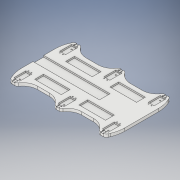
# Autodesk Inventor part: Body_Top
Saved by Autodesk Inventor 2017 (Build 210142000, 142)
## iProperties
Created: 2017-01-25
Part Number: Body_Top
Material: PVC, Unplasticized
Document SubType Name: Modeling
Designer: Alexander Miller
Density: 1.29 g/cm^3
Appearance: Smooth - White
material_thickness: 5,000 mm
body_width: 165,000 mm
leg_distance: 120,000 mm
Author: Alexander Miller
Autodesk Inventor part; units mm, degrees
ref_plane "YZ Plane" through (0, 0, 0) normal (1, 0, 0) x (0, 1, 0)
ref_plane "XZ Plane" through (0, 0, 0) normal (0, 1, 0) x (-1, 0, 0)
ref_plane "XY Plane" through (0, 0, 0) normal (0, 0, 1) x (1, 0, 0)
sketch "Sketch1" plane through (0, 0, 0) normal (0, 1, 0) x (-1, 0, 0)
  line L0 (-175, 0) -> (-175, -82.5)
  line L1 (-175, -82.5) -> (-165, -82.5)
  line L2 (-165, -82.5) -> (-165, -109.25)
  line L3 (-165, -109.25) -> (-135, -109.25)
  line L4 (-135, -109.25) -> (-135, -82.5)
  line L5 (-135, -82.5) -> (-15, -82.5)
  line L6 (-15, -82.5) -> (-15, -109.25)
  line L7 (-15, -109.25) -> (15, -109.25)
  line L8 (15, -109.25) -> (15, -82.5)
  line L9 (15, -82.5) -> (135, -82.5)
  line L10 (135, -82.5) -> (135, -109.25)
  line L11 (135, -109.25) -> (165, -109.25)
  line L12 (165, -109.25) -> (165, -82.5)
  line L13 (165, -82.5) -> (175, -82.5)
  line L14 (175, -82.5) -> (175, 0)
  line L15 (245, 0) -> (-245, 0) projected
  line L16 (-175, 0) -> (-175, 82.5)
  line L17 (-175, 82.5) -> (-165, 82.5)
  line L18 (-165, 82.5) -> (-165, 109.25)
  line L19 (-165, 109.25) -> (-135, 109.25)
  line L20 (-135, 109.25) -> (-135, 82.5)
  line L21 (-135, 82.5) -> (-15, 82.5)
  line L22 (-15, 82.5) -> (-15, 109.25)
  line L23 (-15, 109.25) -> (15, 109.25)
  line L24 (15, 109.25) -> (15, 82.5)
  line L25 (15, 82.5) -> (135, 82.5)
  line L26 (135, 82.5) -> (135, 109.25)
  line L27 (135, 109.25) -> (165, 109.25)
  line L28 (165, 109.25) -> (165, 82.5)
  line L29 (165, 82.5) -> (175, 82.5)
  line L30 (175, 82.5) -> (175, 0)
  point P0 (0, 0)
  point P1 (0, -109.25)
  dimension "d0" = 30
  dimension "d1" = 82.5
  dimension "d2" = 26.75
  dimension "d3" = 10
  dimension "d4" = 120
  constraints: 60 end point, 18 point on line, 14 symmetric about line, 9 perpendicular, 5 equal length, 2 vertical, 1 horizontal alignment, 1 midpoint, 1 vertical alignment
  measures "d0" distance of L10.end L11.end
  measures "d1" distance of L13.end L14.end
  measures "d2" distance of L11.end L12.end
  measures "d3" distance of L12.end L13.end
  measures "d4" distance of L8.end L9.end
extrude "Extrusion1" add sketch "Sketch1" along normal blind 10
sketch "Sketch2" plane through (0, 10, 0) normal (0, 1, 0) x (1, 0, 0)
  line L0 (-140, 57.25) -> (-160, 57.25)
  line L1 (-160, 57.25) -> (-160, 97.75)
  line L2 (-160, 97.75) -> (-140, 97.75)
  line L3 (-140, 97.75) -> (-140, 57.25)
  line L4 (10, 57.25) -> (-10, 57.25)
  line L5 (-10, 57.25) -> (-10, 97.75)
  line L6 (-10, 97.75) -> (10, 97.75)
  line L7 (10, 97.75) -> (10, 57.25)
  line L8 (160, 57.25) -> (140, 57.25)
  line L9 (140, 57.25) -> (140, 97.75)
  line L10 (140, 97.75) -> (160, 97.75)
  line L11 (160, 97.75) -> (160, 57.25)
  line L12 (-245, 0) -> (245, 0) projected
  line L13 (-140, -57.25) -> (-160, -57.25)
  line L14 (-160, -57.25) -> (-160, -97.75)
  line L15 (-160, -97.75) -> (-140, -97.75)
  line L16 (-140, -97.75) -> (-140, -57.25)
  line L17 (10, -57.25) -> (-10, -57.25)
  line L18 (-10, -57.25) -> (-10, -97.75)
  line L19 (-10, -97.75) -> (10, -97.75)
  line L20 (10, -97.75) -> (10, -57.25)
  line L21 (160, -57.25) -> (140, -57.25)
  line L22 (140, -57.25) -> (140, -97.75)
  line L23 (140, -97.75) -> (160, -97.75)
  line L24 (160, -97.75) -> (160, -57.25)
  line L25 (-135, 109.25) -> (-165, 109.25) projected
  line L26 (-165, 109.25) -> (-165, 82.5) projected
  line L27 (-15, 109.25) -> (-15, 82.5) projected
  line L28 (135, 109.25) -> (135, 82.5) projected
  point P0 (0, 0)
  dimension "d7" = 11.5
  dimension "d8" = 5
  dimension "d9" = 20
  dimension "d10" = 40.5
  dimension "d11" = 5
  dimension "d12" = 5
  constraints: 48 end point, 12 symmetric about line, 6 parallel, 4 point on line, 3 horizontal, 3 perpendicular, 2 collinear, 2 horizontal alignment
  measures "d7" distance between parallel lines of L2 L25
  measures "d8" distance between parallel lines of L1 L26
  measures "d9" distance of L1.end L2.end
  measures "d10" distance of L2.end L0.start
  measures "d11" distance between parallel lines of L27 L5
  measures "d12" distance between parallel lines of L9 L28
extrude "Extrusion2" cut sketch "Sketch2" against normal blind 5
sketch "Sketch3" plane through (0, 10, 0) normal (0, 1, 0) x (1, 0, 0)
  circle A0 centre (-155, 53.25) radius 2.25 construction
  circle A1 centre (-145, 53.25) radius 2.25 construction
  circle A2 centre (-155, 101.75) radius 2.25 construction
  circle A3 centre (-145, 101.75) radius 2.25 construction
  circle A4 centre (-5, 53.25) radius 2.25 construction
  circle A5 centre (-5, 101.75) radius 2.25 construction
  line L0 (-135, 109.25) -> (-165, 109.25) projected
  line L1 (-160, 97.75) -> (-140, 97.75) projected
  line L2 (-140, 57.25) -> (-160, 57.25) projected
  line L3 (-160, 57.25) -> (-160, 97.75) projected
  line L4 (-140, 97.75) -> (-140, 57.25) projected
  line L5 (-10, 57.25) -> (-10, 97.75) projected
  line L6 (-245, 0) -> (245, 0) projected
  line L7 (0, 152.95) -> (0, -152.95) projected
  circle A6 centre (-155, 53.25) radius 1.5
  circle A7 centre (-145, 53.25) radius 1.5
  circle A8 centre (-155, 101.75) radius 1.5
  circle A9 centre (-145, 101.75) radius 1.5
  circle A10 centre (-5, 53.25) radius 1.5
  circle A11 centre (-5, 101.75) radius 1.5
  circle A12 centre (155, 53.25) radius 1.5
  circle A13 centre (145, 53.25) radius 1.5
  circle A14 centre (155, 101.75) radius 1.5
  circle A15 centre (145, 101.75) radius 1.5
  circle A16 centre (5, 53.25) radius 1.5
  circle A17 centre (5, 101.75) radius 1.5
  circle A18 centre (-155, -53.25) radius 1.5
  circle A19 centre (-145, -53.25) radius 1.5
  circle A20 centre (-155, -101.75) radius 1.5
  circle A21 centre (-145, -101.75) radius 1.5
  circle A22 centre (-5, -53.25) radius 1.5
  circle A23 centre (-5, -101.75) radius 1.5
  circle A24 centre (155, -53.25) radius 1.5
  circle A25 centre (145, -53.25) radius 1.5
  circle A26 centre (155, -101.75) radius 1.5
  circle A27 centre (145, -101.75) radius 1.5
  circle A28 centre (5, -53.25) radius 1.5
  circle A29 centre (5, -101.75) radius 1.5
  point P0 (0, 0)
  dimension "d17" = 4
  dimension "d18" = 4
  dimension "d19" = 4.5
  dimension "d25" = 2.75
  dimension "d26" = 2.75
  dimension "d27" = 2.75
  dimension "d70" = 3
  constraints: 30 centre point, 18 symmetric about line, 10 equal radius, 6 concentric, 4 horizontal alignment, 3 vertical alignment, 18 other
  measures "d17" distance from line of L1 A2.centre
  measures "d18" distance from line of L2 A0.centre
  measures "d19" diameter of A2
  measures "d25" distance edge to line of A2 L3
  measures "d26" distance edge to line of A3 L4
  measures "d27" distance edge to line of A5 L5
  measures "d70" diameter of A8
extrude "Extrusion3" cut sketch "Sketch3" against normal through all contours A6 | A7 | A8 | A9 | A10 | A11 | A12 | A13 | A14 | A15 | A16 | A17 | A18 | A19 | A20 | A21 | A22 | A23 | A24 | A25 | A26 | A27 | A28 | A29
fillet "Fillet1" radius 10 12 edges at (-165, 5, 109.25) (-135, 5, 109.25) (-15, 5, 109.25) (15, 5, 109.25) (135, 5, 109.25) (165, 5, 109.25) (165, 5, -109.25) (135, 5, -109.25) (15, 5, -109.25) (-15, 5, -109.25) (-135, 5, -109.25) (-165, 5, -109.25)
fillet "Fillet2" radius 50 8 edges at (-135, 5, 82.5) (-15, 5, 82.5) (15, 5, 82.5) (135, 5, 82.5) (135, 5, -82.5) (15, 5, -82.5) (-15, 5, -82.5) (-135, 5, -82.5)
fillet "Fillet3" radius 100 8 edges at (-175, 5, 82.5) (-165, 5, 82.5) (165, 5, 82.5) (175, 5, 82.5) (175, 5, -82.5) (165, 5, -82.5) (-165, 5, -82.5) (-175, 5, -82.5)
sketch "Sketch10" plane through (0, 0, 0) normal (0, -1, 0) x (1, 0, 0)
  circle A0 centre (-150, 87.75) radius 2
  circle A1 centre (0, 87.75) radius 2
  circle A2 centre (150, 87.75) radius 2
  line L0 (-140, 97.75) -> (-160, 97.75) projected
  line L1 (10, 97.75) -> (-10, 97.75) projected
  line L2 (160, 97.75) -> (140, 97.75) projected
  line L3 (-245, 0) -> (245, 0) projected
  circle A3 centre (-150, -87.75) radius 2
  circle A4 centre (0, -87.75) radius 2
  circle A5 centre (150, -87.75) radius 2
  point P0 (0, 0)
  point P1 (-150, 97.75)
  point P2 (0, 97.75)
  point P3 (150, 97.75)
  dimension "d75" = 10
  dimension "d76" = 4
  constraints: 6 centre point, 3 midpoint, 3 symmetric about line, 3 vertical alignment, 2 equal radius, 2 horizontal alignment, 3 other
  measures "d75" distance from line of A0.centre L0
  measures "d76" diameter of A0
extrude "Extrusion10" cut sketch "Sketch10" against normal through all
sketch "Sketch11" plane through (0, 10, 0) normal (0, 1, 0) x (1, 0, 0)
  line L0 (-153.75, 97.75) -> (-146.25, 97.75)
  line L1 (-146.25, 97.75) -> (-146.25, 109.25)
  line L2 (-146.25, 109.25) -> (-153.75, 109.25)
  line L3 (-153.75, 109.25) -> (-153.75, 97.75)
  line L4 (-160, 97.75) -> (-140, 97.75) projected
  line L5 (-140, 57.25) -> (-160, 57.25) projected
  line L6 (-145, 109.25) -> (-155, 109.25) projected
  line L7 (3.75, 97.75) -> (-3.75, 97.75)
  line L8 (-3.75, 97.75) -> (-3.75, 109.25)
  line L9 (-3.75, 109.25) -> (3.75, 109.25)
  line L10 (3.75, 109.25) -> (3.75, 97.75)
  line L11 (153.75, 97.75) -> (146.25, 97.75)
  line L12 (146.25, 97.75) -> (146.25, 109.25)
  line L13 (146.25, 109.25) -> (153.75, 109.25)
  line L14 (153.75, 109.25) -> (153.75, 97.75)
  line L15 (-10, 97.75) -> (10, 97.75) projected
  line L16 (5, 109.25) -> (-5, 109.25) projected
  line L17 (140, 97.75) -> (160, 97.75) projected
  line L18 (155, 109.25) -> (145, 109.25) projected
  line L19 (-245, 0) -> (245, 0) projected
  line L20 (-153.75, -97.75) -> (-146.25, -97.75)
  line L21 (-146.25, -97.75) -> (-146.25, -109.25)
  line L22 (-146.25, -109.25) -> (-153.75, -109.25)
  line L23 (-153.75, -109.25) -> (-153.75, -97.75)
  line L24 (3.75, -97.75) -> (-3.75, -97.75)
  line L25 (-3.75, -97.75) -> (-3.75, -109.25)
  line L26 (-3.75, -109.25) -> (3.75, -109.25)
  line L27 (3.75, -109.25) -> (3.75, -97.75)
  line L28 (153.75, -97.75) -> (146.25, -97.75)
  line L29 (146.25, -97.75) -> (146.25, -109.25)
  line L30 (146.25, -109.25) -> (153.75, -109.25)
  line L31 (153.75, -109.25) -> (153.75, -97.75)
  point P0 (0, 0)
  point P1 (-150, 109.25)
  point P2 (-150, 97.75)
  point P3 (150, 109.25)
  point P4 (150, 97.75)
  point P5 (0, 109.25)
  point P6 (0, 97.75)
  point P7 (-150, -97.75)
  point P8 (150, -109.25)
  point P9 (150, -97.75)
  point P10 (0, -109.25)
  point P11 (0, -97.75)
  dimension "d81" = 7.5
  constraints: 48 end point, 17 symmetric about line, 8 collinear, 6 midpoint, 6 parallel, 3 horizontal, 3 perpendicular, 3 vertical alignment
  measures "d81" distance of L1.end L2.end
extrude "Extrusion11" cut sketch "Sketch11" against normal blind 2
sketch "Sketch12" plane through (0, 10, 0) normal (0, 1, 0) x (1, 0, 0)
  line L0 (50, -18) -> (-175, -18)
  line L1 (-175, -18) -> (-175, 18)
  line L2 (-175, 18) -> (50, 18)
  line L3 (50, 18) -> (50, -18)
  line L4 (-175, 57.3075) -> (-175, -57.3075) projected
  point P0 (0, 0)
  point P1 (50, 0)
  dimension "d84" = 36
  dimension "d85" = 50
  constraints: 8 end point, 2 parallel, 1 collinear, 1 horizontal, 1 horizontal alignment, 1 midpoint, 1 perpendicular
  measures "d84" distance between parallel lines of L2 L0
  measures "d85" distance of point (0, 0) point (50, 0)
extrude "Extrusion12" cut sketch "Sketch12" against normal blind 5
sketch "Sketch13" plane through (0, 10, 0) normal (0, 1, 0) x (1, 0, 0)
  line L0 (-120, -67.5) -> (-30, -67.5)
  line L1 (-30, -67.5) -> (-30, -37.5)
  line L2 (-30, -37.5) -> (-120, -37.5)
  line L3 (-120, -37.5) -> (-120, -67.5)
  line L4 (-120, 37.5) -> (-30, 37.5)
  line L5 (-30, 37.5) -> (-30, 67.5)
  line L6 (-30, 67.5) -> (-120, 67.5)
  line L7 (-120, 67.5) -> (-120, 37.5)
  line L8 (30, -67.5) -> (120, -67.5)
  line L9 (120, -67.5) -> (120, -37.5)
  line L10 (120, -37.5) -> (30, -37.5)
  line L11 (30, -37.5) -> (30, -67.5)
  line L12 (30, 37.5) -> (120, 37.5)
  line L13 (120, 37.5) -> (120, 67.5)
  line L14 (120, 67.5) -> (30, 67.5)
  line L15 (30, 67.5) -> (30, 37.5)
  line L16 (-54.9443, 82.5) -> (-95.0557, 82.5) projected
  line L17 (-95.0557, -82.5) -> (-54.9443, -82.5) projected
  line L18 (95.0557, 82.5) -> (54.9443, 82.5) projected
  point P0 (0, 0)
  point P1 (-75, -67.5)
  point P2 (-75, -82.5)
  point P3 (75, 82.5)
  point P4 (75, 67.5)
  dimension "d88" = 90
  dimension "d89" = 30
  dimension "d90" = 15
  dimension "d91" = 15
  constraints: 32 end point, 10 collinear, 8 parallel, 4 horizontal, 4 midpoint, 4 perpendicular, 2 vertical alignment
  measures "d88" distance of L0.start L0.end
  measures "d89" distance of L0.end L1.end
  measures "d90" distance between parallel lines of L6 L16
  measures "d91" distance between parallel lines of L17 L0
extrude "Extrusion13" cut sketch "Sketch13" against normal blind 5
equation "\"d0\" = servo_depth + 2 * material_thickness"
equation "\"d1\" = 0.5 * body_width"
equation "\"d2\" = 0.5 * servo_width + servo_mount_length"
equation "\"d3\" = 2 * material_thickness"
equation "\"d4\" = leg_distance"
equation "\"d7\" = servo_mount_length + material_thickness"
equation "\"d8\" = material_thickness"
equation "\"d9\" = servo_depth"
equation "\"d10\" = servo_width"
equation "\"d11\" = d8"
equation "\"d12\" = d8"
equation "\"d17\" = servo_mount_length - servo_mount_hole_front_distance"
equation "\"d18\" = d17"
equation "\"d19\" = servo_mount_hole_diameter"
equation "\"d25\" = servo_mount_hole_side_distance"
equation "\"d26\" = d25"
equation "\"d27\" = d25"
equation "\"d28\" = material_thickness"
equation "\"d37\" = 2 * material_thickness"
equation "\"d38\" = 10 * material_thickness"
equation "\"material_thickness\" = 5"
equation "\"body_width\" = 165"
equation "\"leg_distance\" = 120"
equation "\"servo_depth\" = 20"
equation "\"servo_width\" = 40.5"
equation "\"servo_mount_length\" = 6.5"
equation "\"servo_mount_hole_front_distance\" = 2.5"
equation "\"servo_mount_hole_diameter\" = 4.5"
equation "\"servo_mount_hole_side_distance\" = 2.75"
body "Solid1"
